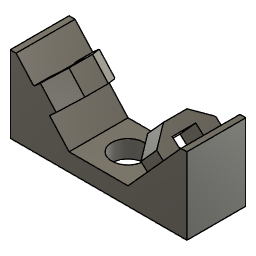
CNC_zip_tie_anchor (Autodesk Fusion 360 design; units mm, degrees)
Autodesk Fusion 360 part; units mm, degrees
note: some values were not read from the file. Chosen so that the rebuilt part matches the saved one: which face or edge a step refers to.
sketch "Sketch1" plane through (0, 0, 0) normal (0, 1, 0) x (1, 0, 0)
  line L0 (15, 5) -> (-15, 5)
  line L1 (-15, 5) -> (-15, -5)
  line L2 (-15, -5) -> (15, -5)
  line L3 (15, -5) -> (15, 5)
  line L4 (15, 5) -> (-15, -5) construction
  line L5 (-15, 5) -> (15, -5) construction
  circle A0 centre (0, 0) radius 2.75
  dimension "d1" = 30
  dimension "d2" = 10
  dimension "d3" = 5.5
  constraint horizontal L0
  constraint perpendicular L0 L1
  constraint parallel L0 L2
  constraint parallel L1 L3
  constraint coincident L4 A0.centre
  constraint coincident L5 A0.centre
  constraint coincident A0.centre origin
  measures "d1" distance of L1.end L2.end
  measures "d2" distance of L0.end L1.end
  measures "d3" diameter of A0
extrude "Extrude1" add sketch "Sketch1" along normal blind 3
sketch "Sketch4" plane through (0, 3, 0) normal (0, 1, 0) x (-1, 0, 0)
  circle A0 centre (0, 0) radius 2.75
  line L0 (-15, 5) -> (-15, -5)
  line L1 (-15, -5) -> (15, -5)
  line L2 (15, -5) -> (15, 5)
  line L3 (15, 5) -> (-15, 5)
  line L4 (-5, -5) -> (5, -5)
  line L5 (5, -5) -> (5, 5)
  line L6 (5, 5) -> (-5, 5)
  line L7 (-5, 5) -> (-5, -5)
  line L8 (-5, -5) -> (5, 5) construction
  line L9 (5, -5) -> (-5, 5) construction
  dimension "d19" = 10
  dimension "d20" = 10
  constraint horizontal L4
  constraint perpendicular L4 L5
  constraint parallel L4 L6
  constraint parallel L5 L7
  constraint coincident L8 A0.centre
  constraint coincident L9 A0.centre
  constraint coincident A0.centre origin
  measures "d19" distance of L5.end L6.end
  measures "d20" distance of L4.start L6.end
extrude "Extrude4" add sketch "Sketch4" along normal blind 10 contours L0 L1 L3 L7 | L1 L2 L3 L5
chamfer "Chamfer3" distance 9 distance2 10 2 edges at (-5, 13, 0) (5, 13, 0) measured on face at (-8.3333, 13, 1.6667) measured on face at (8.3333, 13, -1.6667)
sketch "Sketch5" plane through (-1.2707, -1.1436, 0) normal (0.743294, 0.668965, 0) x (0, 0, -1)
  line L0 (5, 5.5747) -> (5, 19.0283)
  line L1 (5, 19.0283) -> (-5, 19.0283)
  line L2 (-5, 19.0283) -> (-5, 5.5747)
  line L3 (-5, 5.5747) -> (5, 5.5747)
  line L4 (-5, 14.5283) -> (5, 14.5283)
  line L5 (5, 14.5283) -> (5, 10.5283)
  line L6 (5, 10.5283) -> (-5, 10.5283)
  line L7 (-5, 10.5283) -> (-5, 14.5283)
  dimension "d25" = 4
  dimension "d26" = 4.5
  dimension "d27" = 10
  constraint horizontal L4
  constraint vertical L5
  constraint horizontal L6
  constraint vertical L7
  constraint coincident L2 L4.start
  measures "d25" distance of L4.start L6.end
  measures "d26" distance of L1 L4
  measures "d27" distance of L4.start L4.end
extrude "Extrude5" add sketch "Sketch5" along normal blind 4 contours L0 L2 L4 L5 L6 L7
sketch "Sketch6" plane through (1.2707, -1.1436, 0) normal (-0.743294, 0.668965, 0) x (0, 0, 1)
  line L0 (5, 5.5747) -> (5, 19.0283)
  line L1 (5, 19.0283) -> (-5, 19.0283)
  line L2 (-5, 19.0283) -> (-5, 5.5747)
  line L3 (-5, 5.5747) -> (5, 5.5747)
  line L4 (-5, 10.5283) -> (5, 10.5283)
  line L5 (5, 10.5283) -> (5, 14.5283)
  line L6 (5, 14.5283) -> (-5, 14.5283)
  line L7 (-5, 14.5283) -> (-5, 10.5283)
  dimension "d30" = 10
  dimension "d31" = 4.5
  dimension "d32" = 4
  constraint horizontal L4
  constraint vertical L5
  constraint horizontal L6
  constraint vertical L7
  constraint coincident L0 L5.end
  constraint coincident L2 L4.start
  measures "d30" distance of L4.start L4.end
  measures "d31" distance of L1 L6
  measures "d32" distance of L4.start L6.end
extrude "Extrude6" add sketch "Sketch6" along normal blind 4 contours L0 L2 L4 L5 L6 L7
sketch "Sketch7" plane through (-9.7189, 10.7988, 0) normal (-0.668965, 0.743294, 0) x (0, 0, 1)
  line L0 (-5, -1.7096) -> (5, -1.7096)
  line L1 (5, -1.7096) -> (5, 2.2904)
  line L2 (5, 2.2904) -> (-5, 2.2904)
  line L3 (-5, 2.2904) -> (-5, -1.7096)
  line L4 (-2, -1.7096) -> (2, -1.7096)
  line L5 (2, -1.7096) -> (2, 0.2904)
  line L6 (2, 0.2904) -> (-2, 0.2904)
  line L7 (-2, 0.2904) -> (-2, -1.7096)
  dimension "d35" = 4
  dimension "d36" = 2
  dimension "d37" = 3
  constraint horizontal L4
  constraint vertical L5
  constraint horizontal L6
  constraint vertical L7
  constraint coincident L0 L4.start
  measures "d35" distance of L4.start L4.end
  measures "d36" distance of L4.start L6.end
  measures "d37" distance of L3 L7
extrude "Extrude7" cut sketch "Sketch7" against normal blind 4 contours L0 L4 L5 L6 L7
sketch "Sketch8" plane through (9.7189, 10.7988, 0) normal (0.668965, 0.743294, 0) x (0, 0, -1)
  line L0 (-5, -1.7096) -> (5, -1.7096)
  line L1 (5, -1.7096) -> (5, 2.2904)
  line L2 (5, 2.2904) -> (-5, 2.2904)
  line L3 (-5, 2.2904) -> (-5, -1.7096)
  line L4 (-2, -1.7096) -> (2, -1.7096)
  line L5 (2, -1.7096) -> (2, 0.2904)
  line L6 (2, 0.2904) -> (-2, 0.2904)
  line L7 (-2, 0.2904) -> (-2, -1.7096)
  dimension "d40" = 4
  dimension "d41" = 2
  dimension "d42" = 3
  constraint horizontal L4
  constraint vertical L5
  constraint horizontal L6
  constraint vertical L7
  constraint coincident L0 L4.start
  measures "d40" distance of L4.start L4.end
  measures "d41" distance of L4.start L6.end
  measures "d42" distance of L3 L7
extrude "Extrude8" cut sketch "Sketch8" against normal blind 4 contours L0 L4 L5 L6 L7
chamfer "Chamfer4" distance 3 distance2 2.5 4 edges at (6.6786, 10.8444, -5) (6.6786, 10.8444, 5) (-6.6786, 10.8444, -5) (-6.6786, 10.8444, 5) measured on face at (6.2326, 10.3489, -1.6667) measured on face at (6.2326, 10.3489, -1.6667) measured on face at (-7.1245, 11.34, -1.6667) measured on face at (-7.1245, 11.34, -1.6667)
sketch "Sketch2" plane through (0, 1, 0) normal (0, 1, 0) x (-1, 0, 0)
  circle A0 centre (0, 0) radius 2.75
  line L0 (-15, 5) -> (-15, -5)
  line L1 (-15, -5) -> (15, -5)
  line L2 (15, -5) -> (15, 5)
  line L3 (15, 5) -> (-15, 5)
  line L4 (0, -5) -> (0, 5)
  line L5 (-15, 0) -> (15, 0) construction
  line L6 (13, -4) -> (9, -4)
  line L7 (9, -4) -> (9, 4)
  line L8 (9, 4) -> (13, 4)
  line L9 (13, 4) -> (13, -4)
  line L10 (-13, -4) -> (-9, -4)
  line L11 (-9, -4) -> (-9, 4)
  line L12 (-13, 4) -> (-13, -4)
  line L13 (-9, 4) -> (-13, 4)
  dimension "d6" = 8
  dimension "d7" = 4
  dimension "d8" = 4
  dimension "d9" = 2
  constraint midpoint L1 L4.start
  constraint midpoint L3 L4.end
  constraint midpoint L0 L5.start
  constraint midpoint L2 L5.end
  constraint horizontal L6
  constraint vertical L7
  constraint horizontal L8
  constraint vertical L9
  constraint symmetric L4 L6.start L10.start
  constraint symmetric L4 L6.end L10.end
  constraint symmetric L4 L7.end L11.end
  constraint symmetric L4 L8.end L12.start
  measures "d6" distance of L6.end L7.end
  measures "d7" distance of L5 L6
  measures "d8" distance of L6.start L6.end
  measures "d9" distance of L2 L9
extrude "Extrude2" [suppressed]
sketch "Sketch3" plane through (13, 0, 0) normal (1, 0, 0) x (0, 0, -1)
  line L0 (-4, 1) -> (4, 1)
  line L1 (4, 1) -> (4, 4)
  line L2 (4, 4) -> (-4, 4)
  line L3 (-4, 4) -> (-4, 1)
  line L4 (-2, 1) -> (2, 1)
  line L5 (2, 1) -> (2, 2.5)
  line L6 (2, 2.5) -> (-2, 2.5)
  line L7 (-2, 2.5) -> (-2, 1)
  dimension "d12" = 4
  dimension "d13" = 1.5
  dimension "d14" = 2
  constraint horizontal L4
  constraint vertical L5
  constraint horizontal L6
  constraint vertical L7
  constraint coincident L0 L4.start
  measures "d12" distance of L5.end L6.end
  measures "d13" distance of L4.start L6.end
  measures "d14" distance of L3 L7
extrude "Extrude3" [suppressed]
chamfer "Chamfer1" [suppressed]
chamfer "Chamfer2" [suppressed]
